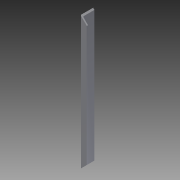
# Autodesk Inventor part: kątownik_mały2
Saved by Autodesk Inventor 2013 (Build 170138000, 138)
## iProperties
Created: 2013-08-20
Part Number: kątownik_mały2
Material: Aluminium 6061
Document SubType Name: Modeling
Designer: Kisieel
Density: 1 g/cm^3
Author: Kisieel
Autodesk Inventor part; units mm, degrees
ref_plane "YZ Plane" through (0, 0, 0) normal (1, 0, 0) x (0, 1, 0)
ref_plane "XZ Plane" through (0, 0, 0) normal (0, 1, 0) x (-1, 0, 0)
ref_plane "XY Plane" through (0, 0, 0) normal (0, 0, 1) x (1, 0, 0)
sketch "Szkic1" plane through (0, 0, 0) normal (0, 0, 1) x (1, 0, 0)
  line L0 (-2.2485, 0) -> (12.0414, 0) projected
  line L1 (0, -4.2485) -> (0, 24.0414) projected
  line L2 (10, 0) -> (1, 0)
  line L3 (0, 1) -> (0, 20)
  line L4 (2, 20) -> (2, 3)
  line L5 (3, 2) -> (10, 2)
  line L6 (0, 20) -> (2, 20)
  line L7 (10, 0) -> (10, 2)
  arc A0 (2, 3) -> (3, 2) centre (3, 3) ccw
  arc A1 (0, 1) -> (1, 0) centre (1, 1) ccw
  point P0 (0, 0)
  dimension "d0" = 20
  dimension "d1" = 10
  dimension "d2" = 2
  dimension "d3" = 1
  constraints: 12 end point, 4 point on circle, 4 point on line, 4 tangent, 2 centre point, 1 collinear, 1 equal radius, 1 parallel, 1 perpendicular, 1 other
  measures "d0" distance of point (0, 0) L3.end
  measures "d1" distance from line of L1 L2.start
  measures "d2" distance between parallel lines of L4 L3
  measures "d3" radius of A0
extrude "Wyciągnięcie proste1" add sketch "Szkic1" along normal blind 210 contours A1 L1 L6 L4 A0 L5 L7 L0
sketch "Szkic2" plane through (1, 0, 0) normal (0, -1, 0) x (1, 0, 0)
  line L0 (0, 0) -> (9, 0) projected
  line L1 (9, 0) -> (9, 210) projected
  line L2 (0, 210) -> (9, 210) projected
  line L3 (-1, 0) -> (-1, 210) projected
  line L4 (-1, 210) -> (9, 200)
  line L5 (9, 200) -> (9, 210)
  line L6 (9, 210) -> (-1, 210)
  line L7 (-1, 0) -> (9, 10)
  line L8 (9, 10) -> (9, 0)
  line L9 (9, 0) -> (-1, 0)
  dimension "d6" = 135
  dimension "d7" = 45
  constraints: 12 end point, 3 perpendicular, 2 point on line
  measures "d6" angle of L3 L4
  measures "d7" angle of L0 L7
extrude "Wyciągnięcie proste2" cut sketch "Szkic2" against normal through all contours L9 L7 L1 L0 | L6 L2 L1 L4
